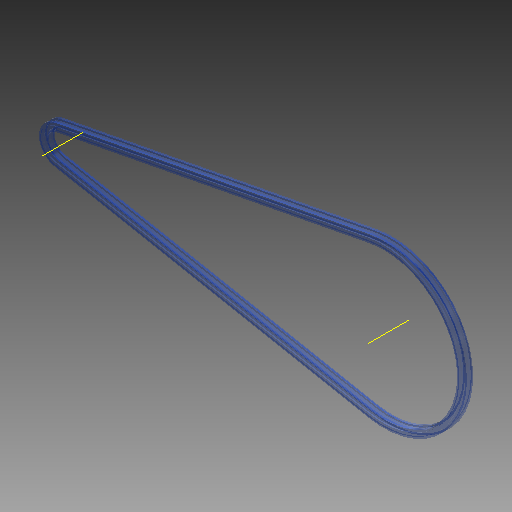
# Autodesk Inventor part: Roller Chain
Saved by Autodesk Inventor 2018.2 (Build 222227000, 227)
## iProperties
Created: 2018-02-07
Part Number: Roller Chain
Material: Generic
Document SubType Name: Modeling
Designer: steele
Density: 1 g/cm^3
Appearance: Clear - Blue
CustomPartVersion: 1
Author: steele
Autodesk Inventor part; units mm, degrees
ref_plane "YZ Plane" through (0, 0, 0) normal (1, 0, 0) x (0, 1, 0)
ref_plane "XZ Plane" through (0, 0, 0) normal (0, 1, 0) x (-1, 0, 0)
ref_plane "XY Plane" through (0, 0, 0) normal (0, 0, 1) x (1, 0, 0)
ref_plane "Work Plane2" through (-383.5917, -0.0109, 0) normal (-1, 0, 0) x (0, 0, 1)
ref_plane "Work Plane3" through (0, 0, 0) normal (-0.9945195, -0.104551, 0) x (0, 0, 1)
sketch "Path" plane through (0, 0, 0) normal (0, 0, 1) x (1, 0, 0)
  arc A0 (-387.0747, 18.0574) -> (-387.0737, -18.0793) centre (-383.5917, -0.0109) ccw
  arc A1 (-17.2197, -89.3545) -> (-17.2247, 89.3536) centre (0, 0) ccw
  line L0 (-17.2197, -89.3545) -> (-387.0737, -18.0793)
  line L1 (-387.0747, 18.0574) -> (-17.2247, 89.3536)
  dimension "d31" = 8.9916
  constraints: 4 end point, 4 point on circle, 2 centre point
ref_plane "Section Plane" through (-387.0737, -18.0793, 0) normal (0.9819328, -0.18923, 0) x (0, 0, 1)
sketch "Section Sketch" plane through (-387.0737, -18.0793, 0) normal (0.9819328, -0.18923, 0) x (0, 0, 1)
  line L0 (-6.35, -1.7907) -> (6.35, -1.7907)
  line L1 (6.35, -1.7907) -> (6.35, 1.7907)
  line L2 (6.35, 1.7907) -> (-6.35, 1.7907)
  line L3 (-6.35, 1.7907) -> (-6.35, -1.7907)
  line L4 (-2.3876, -2.54) -> (2.3876, -2.54)
  line L5 (2.3876, -2.54) -> (2.3876, 2.54)
  line L6 (2.3876, 2.54) -> (-2.3876, 2.54)
  line L7 (-2.3876, 2.54) -> (-2.3876, -2.54)
  line L8 (-2.3876, 0) -> (2.3876, 0) construction
  line L9 (-4.9276, -4.4958) -> (-2.3876, -4.4958)
  line L10 (-2.3876, -4.4958) -> (-2.3876, 4.4958)
  line L11 (-2.3876, 4.4958) -> (-4.9276, 4.4958)
  line L12 (-4.9276, 4.4958) -> (-4.9276, -4.4958)
  line L13 (2.3876, -4.4958) -> (4.9276, -4.4958)
  line L14 (4.9276, -4.4958) -> (4.9276, 4.4958)
  line L15 (4.9276, 4.4958) -> (2.3876, 4.4958)
  line L16 (2.3876, 4.4958) -> (2.3876, -4.4958)
  line L17 (-6.35, 0) -> (6.35, 0) construction
  point P0 (0, 0)
  point P1 (0, 0)
  dimension "d21" = 3.5814
  dimension "d22" = 5.08
  dimension "d23" = 4.7752
  dimension "d24" = 2.54
  dimension "d31" = 8.9916
  dimension "d32" = 12.7
  constraints: 36 end point, 8 midpoint, 8 parallel, 4 horizontal, 4 perpendicular, 3 collinear, 1 coincident, 1 other
  measures "d21" distance between parallel lines of L2 L0
  measures "d22" distance between parallel lines of L6 L4
  measures "d23" distance between parallel lines of L5 L7
  measures "d24" distance between parallel lines of L12 L10
  measures "d31" distance between parallel lines of L11 L9
  measures "d32" distance between parallel lines of L1 L3
sweep "Solid" add profiles "Section Sketch" path "Path" path curves L1 A1 L0 A0
pattern_of_one "Strand Pattern"
equation "\"d21\" = da_d2"
equation "\"d22\" = da_d1"
equation "\"d23\" = da_b1"
equation "\"d24\" = da_t1 + da_t2"
equation "\"d30\" = da_pt"
equation "\"da_p\" = 9.525"
equation "\"da_b1\" = 4.7752"
equation "\"da_h2\" = 8.9916"
equation "\"da_h3\" = 7.7978"
equation "\"da_d1\" = 5.08"
equation "\"da_d2\" = 3.5814"
equation "\"da_pt\" = 10.1346"
equation "\"da_b\" = 12.7"
equation "\"da_t1\" = 1.27"
equation "\"da_t2\" = 1.27"
body "Solid1"
